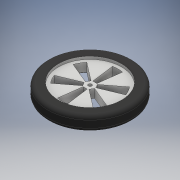
# Autodesk Inventor part: 12 in Wheel
Saved by Autodesk Inventor 2017 (Build 210142000, 142)
## iProperties
Created: 2019-11-18
Part Number: 12 in Wheel
Material: Generic
Document SubType Name: Modeling
Designer: Dell
Density: 1 g/cm^3
Appearance: Default
Author: Dell
Autodesk Inventor part; units mm, degrees
ref_plane "YZ Plane" through (0, 0, 0) normal (1, 0, 0) x (0, 1, 0)
ref_plane "XZ Plane" through (0, 0, 0) normal (0, 1, 0) x (-1, 0, 0)
ref_plane "XY Plane" through (0, 0, 0) normal (0, 0, 1) x (1, 0, 0)
sketch "Sketch1" plane through (0, 0, 0) normal (0, 0, 1) x (1, 0, 0)
  circle A0 centre (0, 0) radius 152.4
  circle A1 centre (0, 0) radius 6.35
  dimension "d0" = 304.8
  dimension "d1" = 12.7
  constraints: 2 centre point, 2 coincident
  measures "d0" diameter of A0
  measures "d1" diameter of A1
extrude "Extrusion1" add sketch "Sketch1" along normal blind 50.8
sketch "Sketch2" plane through (0, 0, 50.8) normal (0, 0, 1) x (1, 0, 0)
  circle A0 centre (0, 0) radius 6.35 projected
  circle A1 centre (0, 0) radius 19.05 construction
  circle A2 centre (0, 0) radius 101.6 construction
  line L0 (7.5, -17.5115) -> (18.3505, -99.9291)
  line L1 (-7.5, -17.5115) -> (-18.3505, -99.9291)
  line L2 (7.5, -17.5115) -> (-7.5, -17.5115)
  arc A3 (-18.3505, -99.9291) -> (18.3505, -99.9291) centre (0, 0) ccw
  arc A4 (-7.5, -17.5115) -> (7.5, -17.5115) centre (0, 0) ccw
  circle A5 centre (0, 0) radius 19.05 construction
  circle A6 centre (0, 0) radius 101.6 construction
  line L3 (18.9154, -2.2606) -> (95.7164, -34.0726)
  line L4 (11.4154, -15.2509) -> (77.3659, -65.8565)
  line L5 (18.9154, -2.2606) -> (11.4154, -15.2509)
  arc A7 (77.3659, -65.8565) -> (95.7164, -34.0726) centre (0, 0) ccw
  arc A8 (11.4154, -15.2509) -> (18.9154, -2.2606) centre (0, 0) ccw
  circle A9 centre (0, 0) radius 19.05 construction
  circle A10 centre (0, 0) radius 101.6 construction
  line L6 (11.4154, 15.2509) -> (77.3659, 65.8565)
  line L7 (18.9154, 2.2606) -> (95.7164, 34.0726)
  line L8 (11.4154, 15.2509) -> (18.9154, 2.2606)
  arc A11 (95.7164, 34.0726) -> (77.3659, 65.8565) centre (0, 0) ccw
  arc A12 (18.9154, 2.2606) -> (11.4154, 15.2509) centre (0, 0) ccw
  circle A13 centre (0, 0) radius 19.05 construction
  circle A14 centre (0, 0) radius 101.6 construction
  line L9 (-7.5, 17.5115) -> (-18.3505, 99.9291)
  line L10 (7.5, 17.5115) -> (18.3505, 99.9291)
  line L11 (-7.5, 17.5115) -> (7.5, 17.5115)
  arc A15 (18.3505, 99.9291) -> (-18.3505, 99.9291) centre (0, 0) ccw
  arc A16 (7.5, 17.5115) -> (-7.5, 17.5115) centre (0, 0) ccw
  circle A17 centre (0, 0) radius 19.05 construction
  circle A18 centre (0, 0) radius 101.6 construction
  line L12 (-18.9154, 2.2606) -> (-95.7164, 34.0726)
  line L13 (-11.4154, 15.2509) -> (-77.3659, 65.8565)
  line L14 (-18.9154, 2.2606) -> (-11.4154, 15.2509)
  arc A19 (-77.3659, 65.8565) -> (-95.7164, 34.0726) centre (0, 0) ccw
  arc A20 (-11.4154, 15.2509) -> (-18.9154, 2.2606) centre (0, 0) ccw
  circle A21 centre (0, 0) radius 19.05 construction
  circle A22 centre (0, 0) radius 101.6 construction
  line L15 (-11.4154, -15.2509) -> (-77.3659, -65.8565)
  line L16 (-18.9154, -2.2606) -> (-95.7164, -34.0726)
  line L17 (-11.4154, -15.2509) -> (-18.9154, -2.2606)
  arc A23 (-95.7164, -34.0726) -> (-77.3659, -65.8565) centre (0, 0) ccw
  arc A24 (-18.9154, -2.2606) -> (-11.4154, -15.2509) centre (0, 0) ccw
  point P0 (0, -17.5115)
  point P1 (0, -101.6)
  point P2 (15.1654, -8.7557)
  point P3 (87.9882, -50.8)
  point P4 (15.1654, 8.7557)
  point P5 (87.9882, 50.8)
  point P6 (0, 17.5115)
  point P7 (0, 101.6)
  point P8 (-15.1654, 8.7557)
  point P9 (-87.9882, 50.8)
  point P10 (-15.1654, -8.7557)
  point P11 (-87.9882, -50.8)
  dimension "d4" = 15
  dimension "d5" = 15
  dimension "d6" = 38.1
  dimension "d7" = 203.2
  dimension "d10" = 360
  constraints: 49 point on circle, 36 end point, 24 centre point, 7 coincident, 2 concentric, 2 vertical alignment, 1 horizontal, 1 midpoint, 103 other
  measures "d4" angle of L0 L1
  measures "d5" distance of L0.start L1.start
  measures "d6" diameter of A1
  measures "d7" diameter of A2
extrude "Extrusion2" cut sketch "Sketch2" against normal through all
sketch "Sketch3" plane through (0, 0, 50.8) normal (0, 0, 1) x (1, 0, 0)
  circle A0 centre (0, 0) radius 114.3
  dimension "d14" = 228.6
  constraints: 1 centre point, 1 coincident
  measures "d14" diameter of A0
extrude "Extrusion3" cut sketch "Sketch3" against normal blind 10
sketch "Sketch4" plane through (0, 0, 0) normal (0, 0, -1) x (-1, 0, 0)
  line L0 (77.3659, -65.8565) -> (11.4154, -15.2509) projected
  arc A0 (77.3659, -65.8565) -> (95.7164, -34.0726) centre (0, 0) ccw projected
  line L1 (18.9154, -2.2606) -> (95.7164, -34.0726) projected
  line L2 (11.4154, -15.2509) -> (18.9154, -2.2606) projected
  line L3 (18.3505, 99.9291) -> (7.5, 17.5115) projected
  arc A1 (18.3505, 99.9291) -> (-18.3505, 99.9291) centre (0, 0) ccw projected
  line L4 (-7.5, 17.5115) -> (-18.3505, 99.9291) projected
  line L5 (7.5, 17.5115) -> (-7.5, 17.5115) projected
  line L6 (-95.7164, -34.0726) -> (-18.9154, -2.2606) projected
  arc A2 (-95.7164, -34.0726) -> (-77.3659, -65.8565) centre (0, 0) ccw projected
  line L7 (-11.4154, -15.2509) -> (-77.3659, -65.8565) projected
  line L8 (-18.9154, -2.2606) -> (-11.4154, -15.2509) projected
  line L9 (-18.3505, -99.9291) -> (-7.5, -17.5115) projected
  arc A3 (-18.3505, -99.9291) -> (18.3505, -99.9291) centre (0, 0) ccw projected
  line L10 (7.5, -17.5115) -> (18.3505, -99.9291) projected
  line L11 (-7.5, -17.5115) -> (7.5, -17.5115) projected
  line L12 (-77.3659, 65.8565) -> (-11.4154, 15.2509) projected
  arc A4 (-77.3659, 65.8565) -> (-95.7164, 34.0726) centre (0, 0) ccw projected
  line L13 (-18.9154, 2.2606) -> (-95.7164, 34.0726) projected
  line L14 (-11.4154, 15.2509) -> (-18.9154, 2.2606) projected
  line L15 (95.7164, 34.0726) -> (18.9154, 2.2606) projected
  arc A5 (95.7164, 34.0726) -> (77.3659, 65.8565) centre (0, 0) ccw projected
  line L16 (11.4154, 15.2509) -> (77.3659, 65.8565) projected
  line L17 (18.9154, 2.2606) -> (11.4154, 15.2509) projected
  circle A6 centre (0, 0) radius 6.35 projected
  circle A7 centre (0, 0) radius 114.3 projected
extrude "Extrusion4" cut sketch "Sketch4" against normal blind 10 contours L0 L2 L1 A0 | L3 L5 L4 A1 | L6 L8 L7 A2 | L9 L11 L10 A3 | L12 L14 L13 A4 | L15 L17 L16 A5 | A6 | A7
fillet "Fillet1" radius 12.7 2 edges at (-152.4, 0, 0) (-152.4, 0, 50.8)
body "Solid1"
